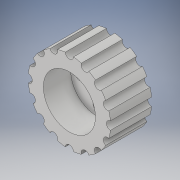
# Autodesk Inventor part: Wheel
Saved by Autodesk Inventor 2017 SP1 (Build 210196100, 196)
## iProperties
Created: 2017-02-11
Part Number: Wheel
Material: Generic
Document SubType Name: Modeling
Designer: Me
Density: 1 g/cm^3
Appearance: Default
Author: Me
Autodesk Inventor part; units mm, degrees
ref_plane "YZ Plane" through (0, 0, 0) normal (1, 0, 0) x (0, 1, 0)
ref_plane "XZ Plane" through (0, 0, 0) normal (0, 1, 0) x (-1, 0, 0)
ref_plane "XY Plane" through (0, 0, 0) normal (0, 0, 1) x (1, 0, 0)
sketch "Sketch1" plane through (0, 0, 0) normal (0, 0, 1) x (1, 0, 0)
  circle A0 centre (0, 0) radius 9.5
  circle A1 centre (0, 6.35) radius 1.425
  circle A2 centre (6.35, 0) radius 1.425
  circle A3 centre (0, -6.35) radius 1.425
  circle A4 centre (-6.35, 0) radius 1.425
  circle A5 centre (0, 0) radius 2
  dimension "d0" = 19
  dimension "d1" = 2.85
  dimension "d2" = 2.85
  dimension "d3" = 2.85
  dimension "d4" = 2.85
  dimension "d5" = 4
  dimension "d6" = 6.35
  dimension "d7" = 6.35
  dimension "d8" = 6.35
  dimension "d9" = 6.35
  constraints: 6 centre point, 2 coincident, 2 horizontal alignment, 2 vertical alignment
  measures "d0" diameter of A0
  measures "d1" diameter of A1
  measures "d2" diameter of A2
  measures "d3" diameter of A3
  measures "d4" diameter of A4
  measures "d5" diameter of A5
  measures "d6" distance of A3.centre point (0, 0)
  measures "d7" distance of A2.centre point (0, 0)
  measures "d8" distance of A1.centre point (0, 0)
  measures "d9" distance of point (0, 0) A4.centre
extrude "Extrusion1" add sketch "Sketch1" along normal blind 5
sketch "Sketch2" plane through (0, 0, 0) normal (0, 0, -1) x (-1, 0, 0)
  circle A0 centre (0, 0) radius 9.5
  circle A1 centre (0, 0) radius 15
  dimension "d12" = 19
  dimension "d13" = 30
  constraints: 2 centre point, 2 coincident
  measures "d12" diameter of A0
  measures "d13" diameter of A1
extrude "Extrusion2" add sketch "Sketch2" against normal blind 15
sketch "Sketch4" plane through (0, 0, 15) normal (0, 0, 1) x (1, 0, 0)
  circle A0 centre (0, 15) radius 1.5
  circle A1 centre (0, 0) radius 15 projected
  circle A2 centre (-15, 0) radius 1.5
  circle A3 centre (0, -15) radius 1.5
  circle A4 centre (15, 0) radius 1.5
  circle A5 centre (0, 0) radius 15 projected
  line L0 (-15, 0) -> (15, 0)
  circle A6 centre (10.6066, 10.6066) radius 1.5
  line L1 (10.6066, 10.6066) -> (0, 0)
  line L2 (0, 0) -> (5.7403, 13.8582)
  line L3 (0, 0) -> (13.8582, 5.7403)
  line L4 (0, 0) -> (13.8582, -5.7403)
  line L5 (0, 0) -> (10.6066, -10.6066)
  line L6 (0, 0) -> (5.7403, -13.8582)
  line L7 (0, 0) -> (-5.7403, -13.8582)
  line L8 (0, 0) -> (-10.6066, -10.6066)
  line L9 (0, 0) -> (-13.8582, -5.7403)
  line L10 (0, 15) -> (0, -15)
  line L11 (0, 0) -> (-5.7403, 13.8582)
  line L12 (0, 0) -> (-10.6066, 10.6066)
  line L13 (0, 0) -> (-13.8582, 5.7403)
  circle A7 centre (5.7403, 13.8582) radius 1.5
  circle A8 centre (13.8582, 5.7403) radius 1.5
  circle A9 centre (13.8582, -5.7403) radius 1.5
  circle A10 centre (10.6066, -10.6066) radius 1.5
  circle A11 centre (5.7403, -13.8582) radius 1.5
  circle A12 centre (-5.7403, -13.8582) radius 1.5
  circle A13 centre (-10.6066, -10.6066) radius 1.5
  circle A14 centre (-13.8582, -5.7403) radius 1.5
  circle A15 centre (-13.8582, 5.7403) radius 1.5
  circle A16 centre (-10.6066, 10.6066) radius 1.5
  circle A17 centre (-5.7403, 13.8582) radius 1.5
  dimension "d21" = 3
  dimension "d22" = 3
  dimension "d23" = 3
  dimension "d24" = 3
  dimension "d29" = 3
  dimension "d30" = 22.5
  dimension "d31" = 22.5
  dimension "d32" = 22.5
  dimension "d33" = 22.5
  dimension "d34" = 22.5
  dimension "d35" = 22.5
  dimension "d36" = 22.5
  dimension "d37" = 22.5
  dimension "d38" = 22.5
  dimension "d39" = 22.5
  dimension "d40" = 22.5
  dimension "d41" = 22.5
  dimension "d42" = 3
  dimension "d43" = 3
  dimension "d44" = 3
  dimension "d45" = 3
  dimension "d46" = 3
  dimension "d47" = 3
  dimension "d48" = 3
  dimension "d49" = 3
  dimension "d50" = 3
  dimension "d51" = 3
  dimension "d52" = 3
  constraints: 28 end point, 16 centre point, 11 coincident, 2 horizontal alignment, 2 vertical alignment, 1 horizontal, 1 vertical, 30 other
  measures "d21" diameter of A2
  measures "d22" diameter of A3
  measures "d23" diameter of A4
  measures "d24" diameter of A0
  measures "d29" diameter of A6
  measures "d30" angle of L0 L3
  measures "d31" angle of L3 L1
  measures "d32" angle of L1 L2
  measures "d33" angle of L0 L4
  measures "d34" angle of L4 L5
  measures "d35" angle of L5 L6
  measures "d36" angle of L10 L7
  measures "d37" angle of L7 L8
  measures "d38" angle of L9 L8
  measures "d39" angle of L10 L11
  measures "d40" angle of L11 L12
  measures "d41" angle of L12 L13
  measures "d42" diameter of A9
  measures "d43" diameter of A10
  measures "d44" diameter of A11
  measures "d45" diameter of A12
  measures "d46" diameter of A13
  measures "d47" diameter of A14
  measures "d48" diameter of A15
  measures "d49" diameter of A16
  measures "d50" diameter of A17
  measures "d51" diameter of A7
  measures "d52" diameter of A8
extrude "Extrusion3" cut sketch "Sketch4" against normal through all contours A0 A1 | A1 L10 A0 | A0 L10 A1 | A17 L11 A1 | A1 A17 | A7 A1 | A1 L2 A7 | L11 A17 A1 | A1 A7 L2 | L0 A1 A2 | A2 A1 L0 | L0 A1 A4 | A4 A1 L0 | L1 A1 A6 | A6 A1 L1 | A8 A1 L3 | L3 A1 A8 | A9 A1 L4 | L4 A1 A9 | A10 A1 L5 | L5 A1 A10 | A11 A1 L6 | L6 A1 A11 | A12 A1 L7 | L7 A1 A12 | A13 A1 L8 | L8 A1 A13 | A14 A1 L9 | L9 A1 A14 | L10 A1 A3 | A3 A1 L10 | A16 A1 L12 | L12 A1 A16 | A15 A1 L13 | L13 A1 A15 | A1 A16 | A1 A2 | A4 A1 | A6 A1 | A1 A8 | A1 A9 | A1 A10 | A1 A11 | A1 A12 | A1 A13 | A1 A14 | A3 A1 | A1 A15
equation "\"d2\" = d1"
equation "\"d3\" = d1"
equation "\"d4\" = d1"
equation "\"d7\" = d6"
equation "\"d8\" = d6"
equation "\"d9\" = d7"
equation "\"d22\" = d21"
equation "\"d23\" = d21"
equation "\"d24\" = d21"
equation "\"d29\" = d24"
equation "\"d31\" = d30"
equation "\"d32\" = d30"
equation "\"d33\" = d30"
equation "\"d34\" = d33"
equation "\"d35\" = d34"
equation "\"d36\" = d30"
equation "\"d37\" = d30"
equation "\"d38\" = d30"
equation "\"d39\" = d30"
equation "\"d40\" = d30"
equation "\"d41\" = d30"
equation "\"d42\" = d21"
equation "\"d43\" = d21"
equation "\"d44\" = d21"
equation "\"d45\" = d21"
equation "\"d46\" = d21"
equation "\"d47\" = d21"
equation "\"d48\" = d21"
equation "\"d49\" = d21"
equation "\"d50\" = d21"
equation "\"d51\" = d21"
equation "\"d52\" = d21"
body "Solid1"
